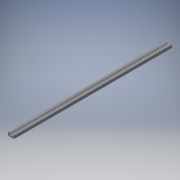
# Autodesk Inventor part: 24in_1050
Saved by Autodesk Inventor 2019 (Build 230136000, 136)
## iProperties
Company: 80/20 Inc.
Created: 2014-04-23
Part Number: 24in_1050
Material: Generic
Document SubType Name: Modeling
Density: 1 g/cm^3
Vendor: 80/20 Inc.
Engineer: Ross Bowman
Designer: Ross Bowman
Catalog Web Link: 8020.net
Appearance: Default
Material: 6105-T5 Aluminum
Author: Ross Bowman
Keywords: 80/20 , 8020 , T-Slot , Extrusion
Autodesk Inventor part; units mm, degrees
ref_plane "YZ Plane" through (0, 0, 0) normal (1, 0, 0) x (0, 1, 0)
ref_plane "XZ Plane" through (0, 0, 0) normal (0, 1, 0) x (-1, 0, 0)
ref_plane "XY Plane" through (0, 0, 0) normal (0, 0, 1) x (1, 0, 0)
sketch "Sketch1" plane through (0, 0, 0) normal (0, 0, 1) x (1, 0, 0)
  circle A0 centre (8.7376, -2.3876) radius 2.032
  circle A1 centre (-8.7376, -2.3876) radius 2.032
  arc A2 (9.5508, 6.3501) -> (10.564, 6.3532) centre (10.0574, 6.3501) ccw
  line L0 (9.5508, 6.3501) -> (6.3306, 6.3501)
  arc A3 (5.3174, 6.3501) -> (6.3306, 6.3501) centre (5.824, 6.3501) ccw
  line L1 (5.3174, 6.3501) -> (4.2872, 6.3501)
  arc A4 (4.2872, 6.3501) -> (3.2382, 5.3011) centre (4.2872, 5.3011) ccw
  line L2 (3.2382, 5.3011) -> (3.2382, 5.1893)
  arc A5 (3.2382, 5.1893) -> (4.2872, 4.1403) centre (4.2872, 5.1893) ccw
  line L3 (4.2872, 4.1403) -> (6.5409, 4.1403)
  arc A6 (7.2003, 2.5463) -> (6.5409, 4.1403) centre (6.5409, 3.2069) ccw
  line L4 (7.2003, 2.5463) -> (3.8742, -0.7738)
  arc A7 (1.6311, -1.7017) -> (3.8742, -0.7738) centre (1.6311, 1.4733) ccw
  line L5 (1.6311, -1.7017) -> (-1.6318, -1.7017)
  arc A8 (-3.8748, -0.7738) -> (-1.6318, -1.7017) centre (-1.6318, 1.4733) ccw
  line L6 (-3.8748, -0.7738) -> (-7.092, 2.4374)
  arc A9 (-6.3875, 4.1403) -> (-7.092, 2.4374) centre (-6.3875, 3.1432) ccw
  line L7 (-6.3875, 4.1403) -> (-4.2879, 4.1403)
  arc A10 (-4.2879, 4.1403) -> (-3.2388, 5.1893) centre (-4.2879, 5.1893) ccw
  line L8 (-3.2388, 5.1893) -> (-3.2388, 5.3011)
  arc A11 (-3.2388, 5.3011) -> (-4.2879, 6.3501) centre (-4.2879, 5.3011) ccw
  line L9 (-4.2879, 6.3501) -> (-5.3196, 6.3501)
  arc A12 (-6.3328, 6.3501) -> (-5.3196, 6.3501) centre (-5.8262, 6.3501) ccw
  line L10 (-6.3328, 6.3501) -> (-9.5528, 6.3501)
  arc A13 (-10.566, 6.3457) -> (-9.5528, 6.3501) centre (-10.0594, 6.3501) ccw
  line L11 (-10.566, 6.3457) -> (-10.5916, 6.3457)
  arc A14 (-10.5916, 6.3457) -> (-12.7, 4.2373) centre (-10.5916, 4.2373) ccw
  line L12 (-12.7, 4.2373) -> (-12.7, -4.2331)
  arc A15 (-12.7, -4.2331) -> (-10.5647, -6.3413) centre (-10.5916, -4.2331) ccw
  arc A16 (-9.5516, -6.35) -> (-10.5647, -6.3413) centre (-10.0581, -6.3412) ccw
  line L13 (-9.5516, -6.35) -> (-6.323, -6.35)
  arc A17 (-5.31, -6.35) -> (-6.323, -6.35) centre (-5.8165, -6.3412) ccw
  line L14 (-5.31, -6.35) -> (5.31, -6.35)
  arc A18 (6.323, -6.35) -> (5.31, -6.35) centre (5.8165, -6.3412) ccw
  line L15 (6.323, -6.35) -> (9.5502, -6.35)
  arc A19 (10.5633, -6.3403) -> (9.5502, -6.35) centre (10.0567, -6.3412) ccw
  line L16 (10.5633, -6.3403) -> (10.589, -6.3404)
  arc A20 (10.589, -6.3404) -> (12.6991, -4.2321) centre (10.5907, -4.2321) ccw
  line L17 (12.6991, -4.2321) -> (12.6991, 4.2448)
  arc A21 (12.6991, 4.2448) -> (10.5907, 6.3532) centre (10.5907, 4.2448) ccw
  line L18 (10.5907, 6.3532) -> (10.564, 6.3532)
  point P0 (0, 0)
  constraints: 40 point on circle, 38 end point, 22 centre point
extrude "Extrusion1" add sketch "Sketch1" against normal blind 609.6
body "Solid1"
